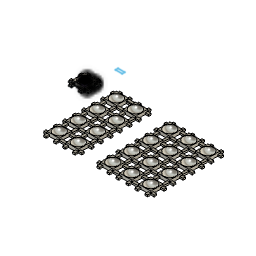
Trays (Autodesk Fusion 360 design; units mm, degrees)
Autodesk Fusion 360 part; units mm, degrees
note: some values were not read from the file. Chosen so that the rebuilt part matches the saved one: which bodies a step acts on.
sketch "Sketch1" plane through (0, 0, 0) normal (0, 0, 1) x (1, 0, 0)
  line L0 (17.5, -17.5) -> (-17.5, -17.5)
  line L1 (-17.5, -17.5) -> (-17.5, 17.5)
  line L2 (-17.5, 17.5) -> (17.5, 17.5)
  line L3 (17.5, 17.5) -> (17.5, -17.5)
  line L4 (17.5, -17.5) -> (-17.5, 17.5) construction
  line L5 (-17.5, -17.5) -> (17.5, 17.5) construction
  line L6 (18.5, -18.5) -> (-18.5, -18.5)
  line L7 (-18.5, -18.5) -> (-18.5, 18.5)
  line L8 (-18.5, 18.5) -> (18.5, 18.5)
  line L9 (18.5, 18.5) -> (18.5, -18.5)
  line L10 (18.5, -18.5) -> (-18.5, 18.5) construction
  line L11 (-18.5, -18.5) -> (18.5, 18.5) construction
  line L12 (0, -18.5) -> (0, 18.5) construction
  line L13 (18.5, 0) -> (-18.5, 0) construction
  line L14 (18.5, -18.5) -> (11, -18.5) construction
  line L15 (11, -18.5) -> (11, -28.5)
  line L16 (11, -28.5) -> (18.5, -28.5)
  line L17 (18.5, -28.5) -> (18.5, -18.5)
  line L18 (-18.5, -18.5) -> (-11, -18.5)
  line L19 (-11, -18.5) -> (-11, -28.5)
  line L20 (-11, -28.5) -> (-18.5, -28.5)
  line L21 (-18.5, -28.5) -> (-18.5, -18.5)
  line L22 (-18.5, -18.5) -> (-28.5, -18.5)
  line L23 (-28.5, -18.5) -> (-28.5, -11)
  line L24 (-28.5, -11) -> (-18.5, -11)
  line L25 (-18.5, -11) -> (-18.5, -18.5)
  line L26 (-18.5, 18.5) -> (-28.5, 18.5)
  line L27 (-28.5, 18.5) -> (-28.5, 11)
  line L28 (-28.5, 11) -> (-18.5, 11)
  line L29 (-18.5, 11) -> (-18.5, 18.5)
  line L30 (18.5, -11) -> (28.5, -11)
  line L31 (28.5, -11) -> (28.5, -18.5)
  line L32 (28.5, -18.5) -> (18.5, -18.5)
  line L33 (18.5, 11) -> (28.5, 11)
  line L34 (28.5, 11) -> (28.5, 18.5)
  line L35 (28.5, 18.5) -> (18.5, 18.5)
  line L36 (18.5, 18.5) -> (18.5, 28.5)
  line L37 (18.5, 28.5) -> (11, 28.5)
  line L38 (11, 28.5) -> (11, 18.5)
  line L39 (-11, 28.5) -> (-11, 18.5)
  line L40 (-18.5, 28.5) -> (-11, 28.5)
  line L41 (-18.5, 18.5) -> (-18.5, 28.5)
  line L42 (18.5, -18.5) -> (-18.5, 18.5) construction
  dimension "d1" = 35
  dimension "d2" = 35
  dimension "d7" = 37
  dimension "d8" = 37
  dimension "d11" = 7.5
  dimension "d12" = 10
  dimension "d13" = 7.5
  dimension "d14" = 10
  dimension "d15" = 10
  dimension "d16" = 7.5
  dimension "d17" = 10
  dimension "d18" = 7.5
  constraint horizontal L0
  constraint perpendicular L0 L1
  constraint parallel L0 L2
  constraint parallel L1 L3
  constraint coincident L4 origin
  constraint coincident L5 origin
  constraint horizontal L6
  constraint perpendicular L6 L7
  constraint parallel L6 L8
  constraint parallel L7 L9
  constraint coincident L10 origin
  constraint coincident L11 origin
  constraint midpoint L6 L12.start
  constraint midpoint L8 L12.end
  constraint midpoint L9 L13.start
  constraint midpoint L7 L13.end
  constraint horizontal L14
  constraint vertical L15
  constraint horizontal L16
  constraint vertical L17
  constraint horizontal L18
  constraint vertical L19
  constraint horizontal L20
  constraint vertical L21
  constraint horizontal L22
  constraint vertical L23
  constraint horizontal L24
  constraint vertical L25
  constraint horizontal L26
  constraint vertical L27
  constraint horizontal L28
  constraint vertical L29
  constraint symmetric L4 L6.start L9.end
  constraint symmetric L4 L6.end L8.end
  constraint symmetric L4 L7.end L8.start
  constraint symmetric L4 L14.end L30.start
  constraint symmetric L4 L15.end L30.end
  constraint symmetric L4 L16.end L31.end
  constraint symmetric L4 L18.end L33.start
  constraint symmetric L4 L19.end L33.end
  constraint symmetric L4 L20.end L34.end
  constraint symmetric L4 L22.end L36.end
  constraint symmetric L4 L23.end L37.end
  constraint symmetric L4 L24.end L38.end
  constraint symmetric L4 L26.end L40.start
  constraint symmetric L4 L27.end L39.start
  constraint symmetric L4 L28.end L39.end
  measures "d1" distance of L1.end L2.end
  measures "d2" distance of L0.end L1.end
  measures "d7" distance of L7.end L8.end
  measures "d8" distance of L6.end L7.end
  measures "d11" distance of L6.start L14.end
  measures "d12" distance of L6.start L16.end
  measures "d13" distance of L6.end L18.end
  measures "d14" distance of L6.end L20.end
  measures "d15" distance of L6.end L22.end
  measures "d16" distance of L6.end L24.end
  measures "d17" distance of L7.end L26.end
  measures "d18" distance of L7.end L28.end
extrude "Extrude1" add sketch "Sketch1" along normal blind 10 contours L0 L1 L2 L3 makes body 1
ref_plane "WorkPlane1" through (0, 0, 20.5) normal (0, 0, 1) x (1, 0, 0)
sphere "SpherePrimitive1" cut diameter 40.25 placed x (1, 0, 0) y (0, 1, 0) z (0, 0, 1) at (0, 0, 20.5) bodies 1
extrude "Extrude2" add sketch "Sketch1" along normal blind 10 separate body contours L6 L7 L8 L9 L18 L25 L29 makes body 2
combine "Combine1" operation add target body 2 tool bodies 1
extrude "Extrude3" add sketch "Sketch1" along normal blind 5 separate body contours L6 L15 L16 L17 | L9 L30 L31 L32 | L6 L18 L19 L20 L21 | L9 L33 L34 L35 | L8 L36 L37 L38 | L7 L26 L27 L28 L29 | L8 L39 L40 L41 makes body 3 at (25.1667, -16, 0) makes body 3 at (13.5, -25.1667, 0) makes body 4 at (21.8333, 16, 0) makes body 4 at (16, 25.1667, 0) makes body 5 at (-16, 21.8333, 0) makes body 5 at (-21.8333, 13.5, 0) makes body 6 at (-13.5, -25.1667, 0)
extrude "Extrude4" add sketch "Sketch1" along normal blind 5 contours L7 L22 L23 L24 L25 bodies 2 6
combine "Combine2" operation add target body 2 tool bodies 3 5 4
copy_body "CopyPasteBodies1" bodies 2 makes body 7
move_body "Move1" bodies 7 to x (1, 0, 0) y (0, 1, 0) z (0, 0, 1) at (95, 0, 0)
copy_body "CopyPasteBodies2" bodies 7 makes body 8
move_body "Move2" bodies 8 to x (1, 0, 0) y (0, 1, 0) z (0, 0, 1) at (0, -57, 0)
copy_body "CopyPasteBodies3" bodies 8 makes body 9
move_body "Move3" bodies 9 to x (1, 0, 0) y (0, 1, 0) z (0, 0, 1) at (0, -57, 0)
copy_body "CopyPasteBodies4" bodies 9 makes body 10
move_body "Move4" bodies 10 to x (1, 0, 0) y (0, 1, 0) z (0, 0, 1) at (0, -57, 0)
combine "Combine3" operation add target body 7 tool bodies 9 8 10
copy_body "CopyPasteBodies5" bodies 7 makes body 11
move_body "Move5" bodies 11 to x (1, 0, 0) y (0, 1, 0) z (0, 0, 1) at (57, 0, 0)
copy_body "CopyPasteBodies6" bodies 7 11 makes body 12 makes body 13
move_body "Move6" bodies 12 13 to x (1, 0, 0) y (0, 1, 0) z (0, 0, 1) at (160, 0, 0)
combine "Combine4" operation add target body 11 tool bodies 7
copy_body "CopyPasteBodies7" bodies 13 makes body 14
move_body "Move7" bodies 14 to x (1, 0, 0) y (0, 1, 0) z (0, 0, 1) at (57, 0, 0)
combine "Combine5" operation add target body 12 tool bodies 13 14
sketch "Sketch3" plane through (0, 0, 0) normal (0, 0, 1) x (1, 0, 0)
  line L0 (10, 90) -> (29.75, 90)
  line L1 (29.75, 90) -> (29.75, 82.5)
  line L2 (29.75, 82.5) -> (10, 82.5)
  line L3 (10, 82.5) -> (10, 90)
  dimension "d23" = 19.75
  dimension "d24" = 7.5
  constraint horizontal L0
  constraint vertical L1
  constraint horizontal L2
  constraint vertical L3
  measures "d23" distance of L0.start L0.end
  measures "d24" distance of L0.start L2.end
extrude "Extrude5" add sketch "Sketch3" along normal blind 3 separate body makes body 15
move_body "Move8" bodies 15 to x (1, 0, 0) y (0, 1, 0) z (0, 0, 1) at (103.625, -71.5, 5)
extrude "Extrude6" add 1 faces at (120.2083, 13.5, 8) along direction (0, 0, 1) blind 2 on bodies 15 bodies 15
extrude "Extrude7" cut 1 faces at (120.2083, 13.5, 10) along direction (0, 0, -1) blind 1 on bodies 15 bodies 15
extrude "Extrude8" cut 1 faces at (120.2083, 13.5, 9) along direction (0, 0, -1) blind 1 on bodies 15 bodies 15
